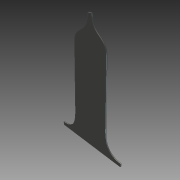
# Autodesk Inventor part: Plate
Saved by Autodesk Inventor 2012 (Build 160160000, 160)
## iProperties
Created: 2013-02-28
Part Number: Plate
Material: High Impact Polystyrene
Document SubType Name: Modeling
Designer: fixer
Mass: 147.124 g
Surface Area: 944.06 cm^2
Volume: 143.957 cm^3
Density: 1.022 g/cm^3
Author: fixer
Autodesk Inventor part; units mm, degrees
ref_plane "YZ Plane" through (0, 0, 0) normal (1, 0, 0) x (0, 1, 0)
ref_plane "XZ Plane" through (0, 0, 0) normal (0, 1, 0) x (-1, 0, 0)
ref_plane "XY Plane" through (0, 0, 0) normal (0, 0, 1) x (1, 0, 0)
sketch "Sketch1" plane through (0, 0, 0) normal (0, 0, 1) x (1, 0, 0)
  line L0 (76.2, -12.7) -> (381, -12.7) construction
  line L1 (-76.2, -12.7) -> (-381, -12.7) construction
  line L2 (-76.2, 0) -> (-381, 0) construction
  line L3 (76.2, 0) -> (381, 0) construction
  line L4 (0, -116.2267) -> (0, 608.4603)
  line L5 (0, -12.7) -> (-122.0009, -12.7)
  line L6 (-122.0009, -12.7) -> (-122.0009, 0)
  line L7 (0, 394.3626) -> (-6.35, 394.3626)
  line L8 (-52.4512, 312.4765) -> (-60.2591, 93.2692)
  spline S0 degree 3 poles (-122.0009, 0) (-64.2705, 0) (-61.6839, 53.2691) (-60.2591, 93.2692) knots 0 0 0 0 1 1 1 1
  line L9 (-127.2981, 0) -> (-116.7037, 0) construction
  arc A0 (-126.2344, 0.0955) -> (-117.7675, 0.0955) centre (-122.0009, 93.8482) ccw construction
  line L10 (52.4512, 312.4765) -> (60.2591, 93.2692)
  line L11 (0, 394.3626) -> (6.35, 394.3626)
  spline S1 degree 3 poles (122.0009, 0) (64.2705, 0) (61.6839, 53.2691) (60.2591, 93.2692) knots 0 0 0 0 1 1 1 1
  line L12 (127.2981, 0) -> (116.7037, 0) construction
  arc A1 (117.7675, 0.0955) -> (126.2344, 0.0955) centre (122.0009, 93.8482) ccw construction
  line L13 (0, -12.7) -> (122.0009, -12.7)
  line L14 (122.0009, -12.7) -> (122.0009, 0)
  spline S2 degree 4 poles (-6.35, 394.3626) (-6.35, 370.6692) (-16.2148, 349.4175) (-49.2512, 345.2253) (-52.0931, 322.5296) (-52.4512, 312.4765) knots 0 0 0 0 0 0.529809 1 1 1 1 1
  line L15 (-6.35, 421.2444) -> (-6.35, 367.4808) construction
  arc A2 (-7.9378, 373.0956) -> (-7.9378, 415.6296) centre (-149.5647, 394.3626) ccw construction
  spline S3 degree 4 poles (6.35, 394.3626) (6.35, 349.6419) (36.5958, 353.9783) (51.6896, 333.8574) (52.4512, 312.4765) knots 0 0 0 0 0 1 1 1 1 1
  line L16 (6.35, 421.2444) -> (6.35, 367.4808) construction
  arc A3 (7.9378, 415.6296) -> (7.9378, 373.0956) centre (149.5647, 394.3626) ccw construction
  line L17 (-23.1287, 353.4652) -> (-48.6526, 335.307) construction
  arc A4 (-25.2872, 350.8986) -> (-45.5201, 336.5045) centre (17.5347, 269.2893) ccw construction
  point P0 (0, 0)
  point P1 (-35.8906, 344.3861)
  point P2 (35.8906, 344.3861)
  dimension "d0" = 6.35
  constraints: 36 end point, 16 symmetric about line, 9 horizontal, 8 midpoint, 5 centre point, 5 point on circle, 5 point on line, 4 vertical, 2 perpendicular, 21 other
  measures "d0" distance of L7.start L7.end
extrude "Extrusion1" add sketch "Sketch1" against normal blind 3.175
body "Solid1"
